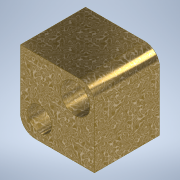
# Autodesk Inventor part: spacer dubbele hoogte behuizing
Saved by Autodesk Inventor 2021 (Build 250183000, 183)
## iProperties
Created: 2023-11-13
Part Number: spacer dubbele hoogte behuizing
Material: Generic
Document SubType Name: Modeling
Designer: Elias
Density: 1 g/cm^3
Appearance: Foil Gold
Author: Elias
Autodesk Inventor part; units mm, degrees
ref_plane "YZ Plane" through (0, 0, 0) normal (1, 0, 0) x (0, 1, 0)
ref_plane "XZ Plane" through (0, 0, 0) normal (0, 1, 0) x (-1, 0, 0)
ref_plane "XY Plane" through (0, 0, 0) normal (0, 0, 1) x (1, 0, 0)
sketch "Sketch1" plane through (0, 0, 0) normal (0, 0, 1) x (1, 0, 0)
  line L0 (5, 0) -> (25, 0)
  line L1 (25, 0) -> (25, 20)
  line L2 (20, 25) -> (0, 25)
  line L3 (0, 25) -> (0, 5)
  arc A0 (25, 20) -> (20, 25) centre (20, 20) ccw
  arc A1 (0, 5) -> (5, 0) centre (5, 5) ccw
  point P0 (0, 0)
  point P1 (25, 25)
  dimension "d0" = 25
  dimension "d1" = 25
  dimension "d2" = 5
  dimension "d29" = 5
  constraints: 8 end point, 4 point on circle, 4 point on line, 4 tangent, 2 centre point, 2 parallel, 1 horizontal, 1 perpendicular
  measures "d0" distance of point (25, 25) L2.end
  measures "d1" distance of L0.end point (25, 25)
  measures "d2" radius of A0
  measures "d29" radius of A1
extrude "Extrusion1" add sketch "Sketch1" along normal blind 22
sketch "Sketch2" plane through (0, 0, 22) normal (0, 0, 1) x (1, 0, 0)
  line L0 (20, 25) -> (0, 25) projected
  line L1 (25, 0) -> (25, 20) projected
  point P0 (0, 0)
  point P1 (18.5, 18.5)
  dimension "d12" = 6.5
  dimension "d13" = 6.5
  measures "d12" distance from line of L0 point (18.5, 18.5)
  measures "d13" distance from line of L1 point (18.5, 18.5)
hole "Hole1" at (18.5, 18.5, 22) direction (0, 0, -1) diameter 10 depth 16
sketch "Sketch3" plane through (18.5, 18.5, 6) normal (0, 0, 1) x (1, 0, 0)
  line L0 (6.5, -18.5) -> (6.5, 1.5) projected
  line L1 (1.5, 6.5) -> (-18.5, 6.5) projected
  point P0 (-18.5, -18.5)
  point P1 (0, 0)
  dimension "d21" = 6.5
  dimension "d22" = 6.5
  measures "d21" distance from line of L0 point (0, 0)
  measures "d22" distance from line of L1 point (0, 0)
hole "Hole2" at (18.5, 18.5, 6) direction (0, 0, -1) diameter 3 depth 15
chamfer "Chamfer2" distance 2 angle 45 1 edges at (18.5, 20, 6)
sketch "Sketch4" plane through (0, 0, 22) normal (0, 0, 1) x (1, 0, 0)
  line L0 (5, 0) -> (25, 0) projected
  line L1 (0, 25) -> (0, 5) projected
  point P0 (0, 0)
  point P1 (6.5, 6.5)
  dimension "d37" = 6.5
  dimension "d38" = 6.5
  measures "d37" distance from line of L0 point (6.5, 6.5)
  measures "d38" distance from line of L1 point (6.5, 6.5)
hole "Hole3" at (6.5, 6.5, 22) direction (0, 0, -1) diameter 8.2 depth 16
body "Solid1"
